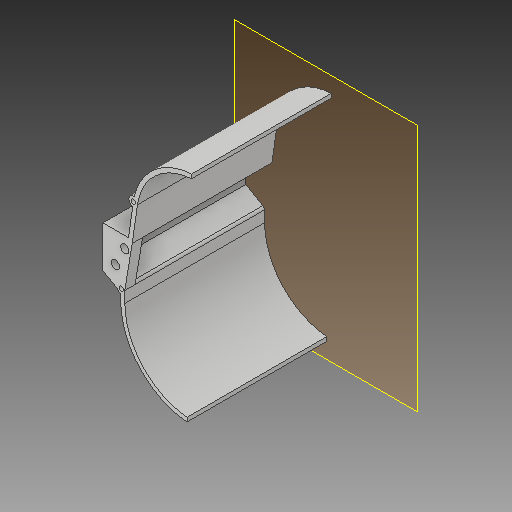
# Autodesk Inventor part: case top half
Saved by Autodesk Inventor 2017 (Build 210142000, 142)
## iProperties
Created: 2018-04-17
Part Number: case top half
Material: Generic
Document SubType Name: Modeling
Designer: RKL
Density: 1 g/cm^3
Appearance: Default
Author: RKL
Autodesk Inventor part; units mm, degrees
ref_plane "YZ Plane" through (0, 0, 0) normal (1, 0, 0) x (0, 1, 0)
ref_plane "XZ Plane" through (0, 0, 0) normal (0, 1, 0) x (-1, 0, 0)
ref_plane "Work Plane1" through (0, 0, 0) normal (0, 0, 1) x (1, 0, 0)
sketch "Sketch1" plane through (0, 0, 0) normal (0, 0, 1) x (1, 0, 0)
  circle A0 centre (-55.8916, -14.7421) radius 1.397 projected
  circle A1 centre (-83.8916, 18.2579) radius 1.397 construction
  circle A2 centre (-83.8916, -14.7421) radius 1.397 construction
  circle A3 centre (-55.8916, 18.2579) radius 1.397 projected
  circle A4 centre (2.1895, 105.4705) radius 2.159 projected
  circle A5 centre (-2.169, -104.4843) radius 2.159 projected
  circle A6 centre (60.6164, 51.7463) radius 2.159 projected
  circle A7 centre (-58.4167, 54.2173) radius 2.159 projected
  arc A8 (6.6818, 105.2084) -> (-2.3099, 105.3951) centre (2.1895, 105.4705) ccw projected
  arc A9 (-2.3099, 105.3951) -> (-57.5952, 58.6417) centre (0.9442, 45.4834) ccw projected
  arc A10 (-57.5952, 58.6417) -> (-59.0718, 49.7652) centre (-58.4167, 54.2173) ccw projected
  line L0 (-59.0718, 49.7652) -> (-63.1925, 21.7579) projected
  line L1 (-87.8916, 21.7579) -> (-63.1925, 21.7579) projected
  line L2 (-87.8916, -18.2421) -> (-87.8916, 21.7579) projected
  line L3 (-87.8916, -18.2421) -> (-74.0344, -26.2425) projected
  arc A11 (-74.0344, -26.2425) -> (-70.4822, -28.7807) centre (-69.9706, -24.3098) ccw projected
  arc A12 (-70.4822, -28.7807) -> (-6.6627, -104.2463) centre (-0.7162, -34.4994) ccw projected
  arc A13 (-6.6627, -104.2463) -> (2.3307, -104.433) centre (-2.169, -104.4843) ccw projected
  arc A14 (2.3307, -104.433) -> (69.2271, -31.6809) centre (-0.7162, -34.4994) ccw projected
  arc A15 (69.2271, -31.6809) -> (68.4317, -22.7173) centre (68.9014, -27.1927) ccw projected
  line L4 (68.4317, -22.7173) -> (61.0862, 47.2708) projected
  arc A16 (61.0862, 47.2708) -> (59.9792, 56.2009) centre (60.6164, 51.7463) ccw projected
  arc A17 (59.9792, 56.2009) -> (6.6818, 105.2084) centre (0.9442, 45.4834) ccw projected
  circle A18 centre (-69.9706, -24.3098) radius 2.159 projected
  circle A19 centre (68.9014, -27.1927) radius 2.159 projected
  circle A20 centre (0.9442, 45.4834) radius 17.5 projected
  circle A21 centre (-0.7162, -34.4994) radius 17.5 projected
  circle A22 centre (-66.7556, 10.6536) radius 4 projected
  circle A23 centre (-75.8916, -7.1378) radius 4 projected
  circle A24 centre (68.9014, -27.1927) radius 2.159 construction
  circle A25 centre (60.6164, 51.7463) radius 2.159 construction
  circle A26 centre (-2.169, -104.4843) radius 2.159 construction
  circle A27 centre (2.1895, 105.4705) radius 2.159 construction
  arc A28 (6.6818, 105.2084) -> (-2.3099, 105.3951) centre (2.1895, 105.4705) ccw construction
  arc A29 (59.9792, 56.2009) -> (6.6818, 105.2084) centre (0.9442, 45.4834) ccw construction
  arc A30 (61.0862, 47.2708) -> (59.9792, 56.2009) centre (60.6164, 51.7463) ccw construction
  line L5 (61.0862, 47.2708) -> (68.4317, -22.7173) construction
  arc A31 (69.2271, -31.6809) -> (68.4317, -22.7173) centre (68.9014, -27.1927) ccw construction
  arc A32 (2.3307, -104.433) -> (69.2271, -31.6809) centre (-0.7162, -34.4994) ccw construction
  arc A33 (-6.6627, -104.2463) -> (2.3307, -104.433) centre (-2.169, -104.4843) ccw construction
  line L6 (-6.6627, -104.2463) -> (-6.5797, -100.2463) construction
  arc A34 (-6.5797, -100.2463) -> (64.9314, -27.6121) centre (-0.7162, -34.4994) ccw construction
  line L7 (64.9314, -27.6121) -> (56.6497, 51.3276) construction
  arc A35 (56.6497, 51.3276) -> (-2.393, 101.3951) centre (0.9442, 45.4834) ccw construction
  line L8 (-2.393, 101.3951) -> (-2.3099, 105.3951) construction
  line L9 (-6.6627, -104.2463) -> (-6.5797, -100.2463)
  line L10 (-2.393, 101.3951) -> (-2.3099, 105.3951)
  arc A36 (-2.393, 101.3951) -> (-54.4704, 53.6367) centre (0.9442, 45.4834) ccw
  line L11 (-54.4704, 53.6367) -> (-59.6022, 18.7579)
  line L12 (-59.6022, 18.7579) -> (-84.8916, 18.7579)
  line L13 (-84.8916, 18.7579) -> (-84.8916, -12.0475)
  arc A37 (-66.7218, -35.0506) -> (-6.5797, -100.2463) centre (-0.7162, -34.4994) ccw
  arc A38 (-66.8117, -24.2835) -> (-68.3911, -21.5741) centre (-69.9706, -24.3098) ccw
  line L14 (-66.7218, -35.0506) -> (-66.8117, -24.2835)
  line L15 (-84.8916, -12.0475) -> (-68.3911, -21.5741)
  point P0 (0, 0)
  dimension "d0" = 1
  dimension "d1" = 3
  dimension "d2" = 3
  constraints: 14 end point, 6 point on circle, 4 parallel, 4 tangent, 3 centre point, 3 coincident, 2 collinear, 1 horizontal
  measures "d0" radial gap between concentric circles of A18 A38
  measures "d1" distance between parallel lines of L2 L13
  measures "d2" distance between parallel lines of L1 L12
extrude "Extrusion1" add sketch "Sketch1" along normal blind 125 contours L10 A36 L11 L12 L13 L15 A38 L14 A37 L9 A12 A11 L3 L2 L1 L0 A10 A9
sketch "Sketch2" plane through (0, 0, 125) normal (0, 0, 1) x (1, 0, 0)
  circle A0 centre (-69.9706, -24.3098) radius 2.159 projected
  circle A1 centre (-58.4167, 54.2173) radius 2.159 projected
  arc A2 (-2.3099, 105.3951) -> (-57.5952, 58.6417) centre (0.9442, 45.4834) ccw projected
  arc A3 (-57.5952, 58.6417) -> (-59.0718, 49.7652) centre (-58.4167, 54.2173) ccw projected
  line L0 (-59.0718, 49.7652) -> (-63.1925, 21.7579) projected
  line L1 (-63.1925, 21.7579) -> (-87.8916, 21.7579) projected
  line L2 (-87.8916, 21.7579) -> (-87.8916, -18.2421) projected
  line L3 (-87.8916, -18.2421) -> (-74.0344, -26.2425) projected
  arc A4 (-74.0344, -26.2425) -> (-70.4822, -28.7807) centre (-69.9706, -24.3098) ccw projected
  arc A5 (-70.4822, -28.7807) -> (-6.6627, -104.2463) centre (-0.7162, -34.4994) ccw projected
  line L4 (-6.6627, -104.2463) -> (-6.5797, -100.2463) projected
  arc A6 (-66.7218, -35.0506) -> (-6.5797, -100.2463) centre (-0.7162, -34.4994) ccw projected
  line L5 (-66.7218, -35.0506) -> (-66.8117, -24.2835) projected
  arc A7 (-66.8117, -24.2835) -> (-68.3911, -21.5741) centre (-69.9706, -24.3098) ccw projected
  line L6 (-68.3911, -21.5741) -> (-84.8916, -12.0475) projected
  line L7 (-84.8916, -12.0475) -> (-84.8916, 18.7579) projected
  line L8 (-84.8916, 18.7579) -> (-59.6022, 18.7579) projected
  line L9 (-59.6022, 18.7579) -> (-54.4704, 53.6367) projected
  arc A8 (-2.393, 101.3951) -> (-54.4704, 53.6367) centre (0.9442, 45.4834) ccw projected
  line L10 (-2.393, 101.3951) -> (-2.3099, 105.3951) projected
  circle A9 centre (-66.7556, 10.6536) radius 4 projected
  circle A10 centre (-75.8916, -7.1378) radius 4 projected
  line L11 (-66.7218, -35.0506) -> (-66.8117, -24.2835) projected
  line L12 (-59.6022, 18.7579) -> (-66.8117, -24.2835)
  point P0 (0, 0)
  constraints: 2 end point
ref_plane "Work Plane2" through (-78.4932, -111.5319, 135) normal (0, 0, -1) x (0, 1, 0)
extrude "Extrusion2" add sketch "Sketch2" along normal up to surface (10 mm away)
body "Solid1"
